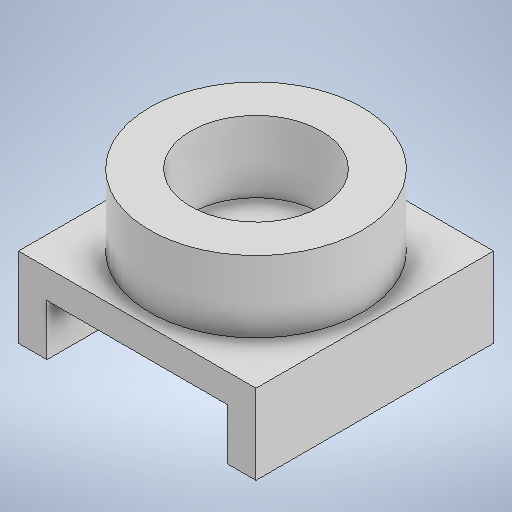
# Autodesk Inventor part: MMAE 232 Assignment 2_Servo Horn 2 - Dylan Tamras
Saved by Autodesk Inventor 2025.2 (Build 292293000, 293)
## iProperties
Created: 2025-01-19
Part Number: MMAE 232 Assignment 2_Servo Horn 2 - Dylan Tamras
Material: Generic
Document SubType Name: Modeling
Designer: Dylan
Density: 1 g/cm^3
Appearance: Default
Author: Dylan
Autodesk Inventor part; units mm, degrees
ref_plane "YZ Plane" through (0, 0, 0) normal (1, 0, 0) x (0, 1, 0)
ref_plane "XZ Plane" through (0, 0, 0) normal (0, 1, 0) x (-1, 0, 0)
ref_plane "XY Plane" through (0, 0, 0) normal (0, 0, 1) x (1, 0, 0)
sketch "Sketch1" plane through (0, 0, 0) normal (0, 1, 0) x (-1, 0, 0)
  line L0 (0, 0) -> (10, 0)
  line L1 (10, 0) -> (10, -10)
  line L2 (10, -10) -> (0, -10)
  line L3 (0, -10) -> (0, 0)
  dimension "d0" = 10
  dimension "d1" = 10
  constraints: 8 end point, 2 parallel, 1 horizontal, 1 perpendicular
  measures "d0" distance of L1.end L2.end
  measures "d1" distance of L0.end L1.end
extrude "Extrusion1" add sketch "Sketch1" along normal blind 3.36
sketch "Sketch2" plane through (0, 3.36, 0) normal (0, 1, 0) x (1, 0, 0)
  line L0 (-10, 10) -> (-10, 0) projected
  circle A0 centre (-5, 5) radius 1.37
  point P0 (0, 0)
  dimension "d4" = 2.74
  constraints: 1 centre point
  measures "d4" diameter of A0
extrude "Extrusion2" cut sketch "Sketch2" against normal blind 3.36
sketch "Sketch3" plane through (0, 3.36, 0) normal (0, 1, 0) x (1, 0, 0)
  line L0 (-10, 10) -> (-10, 0) projected
  circle A0 centre (-5, 5) radius 2.75
  circle A1 centre (-5, 5) radius 4.475
  point P0 (0, 0)
  dimension "d7" = 5.5
  dimension "d8" = 8.95
  constraints: 2 centre point, 1 coincident
  measures "d7" diameter of A0
  measures "d8" diameter of A1
extrude "Extrusion3" add sketch "Sketch3" along normal blind 3
sketch "Sketch4" plane through (0, 0, 0) normal (0, -1, 0) x (1, 0, 0)
  line L0 (-1.2, 0) -> (-1.2, -10)
  line L1 (-8.8, 0) -> (-8.8, -10)
  line L2 (-1.2, -10) -> (-8.8, -10)
  line L3 (0, -10) -> (-10, -10) projected
  line L4 (-8.8, 0) -> (-1.2, 0)
  line L5 (-10, 0) -> (0, 0) projected
  dimension "d11" = 1.2
  constraints: 8 end point, 2 collinear, 1 vertical
  measures "d11" distance of L5.end L0.start
extrude "Extrusion4" cut sketch "Sketch4" against normal blind 2.16
body "Solid1"
